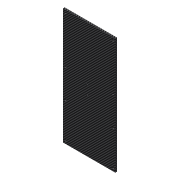
# Autodesk Inventor part: Chassis-2
Saved by Autodesk Inventor 2018 (Build 220112000, 112)
## iProperties
Created: 2018-01-20
Part Number: Chassis-2
Material: CFK
Document SubType Name: Modeling
Designer: fhinstall
Density: 1.43 g/cm^3
Appearance: Kohlenstofffaser
Mass: 68.419 g
Surface Area: 337.638 cm^2
Volume: 47.8454 cm^3
Author: fhinstall
Autodesk Inventor part; units mm, degrees
ref_plane "YZ Plane" through (0, 0, 0) normal (1, 0, 0) x (0, 1, 0)
ref_plane "XZ Plane" through (0, 0, 0) normal (0, 1, 0) x (-1, 0, 0)
ref_plane "XY Plane" through (0, 0, 0) normal (0, 0, 1) x (1, 0, 0)
sketch "Skizze1" plane through (0, 0, 0) normal (0, 1, 0) x (-1, 0, 0)
  line L0 (45, 100) -> (45, -100)
  line L1 (45, -100) -> (-45, -100)
  line L2 (-45, -100) -> (-45, 100)
  line L3 (-45, 100) -> (45, 100)
  line L4 (0, 61.8387) -> (0, -129.7607) construction
  line L5 (83.0665, 0) -> (-88.5254, 0) construction
  circle A0 centre (41, 95) radius 1.7
  circle A1 centre (-41, 95) radius 1.7
  circle A2 centre (-41, -95) radius 1.7
  circle A3 centre (41, -95) radius 1.7
  circle A4 centre (3.1127, 7.2251) radius 1.5558
  circle A5 centre (3.1127, -8.3324) radius 1.5558
  circle A6 centre (-41, 15) radius 1.7
  circle A7 centre (41, 15) radius 1.7
  circle A8 centre (-41, -65) radius 1.7
  circle A9 centre (41, -65) radius 1.7
  circle A10 centre (-41, -145) radius 1.7
  circle A11 centre (41, -145) radius 1.7
  circle A12 centre (-41, -225) radius 1.7
  circle A13 centre (41, -225) radius 1.7
  circle A14 centre (-41, -305) radius 1.7
  circle A15 centre (41, -305) radius 1.7
  circle A16 centre (-41, -385) radius 1.7
  circle A17 centre (41, -385) radius 1.7
  circle A18 centre (-41, -465) radius 1.7
  circle A19 centre (41, -465) radius 1.7
  circle A20 centre (-41, -545) radius 1.7
  circle A21 centre (41, -545) radius 1.7
  circle A22 centre (-41, -625) radius 1.7
  circle A23 centre (41, -625) radius 1.7
  circle A24 centre (-41, -705) radius 1.7
  circle A25 centre (41, -705) radius 1.7
  circle A26 centre (-41, -785) radius 1.7
  circle A27 centre (41, -785) radius 1.7
  circle A28 centre (-41, -865) radius 1.7
  circle A29 centre (41, -865) radius 1.7
  circle A30 centre (-41, -945) radius 1.7
  circle A31 centre (41, -945) radius 1.7
  circle A32 centre (-41, -1025) radius 1.7
  circle A33 centre (41, -1025) radius 1.7
  circle A34 centre (-41, -1105) radius 1.7
  circle A35 centre (41, -1105) radius 1.7
  circle A36 centre (-41, -1185) radius 1.7
  circle A37 centre (41, -1185) radius 1.7
  circle A38 centre (-41, -1265) radius 1.7
  circle A39 centre (41, -1265) radius 1.7
  circle A40 centre (-41, -1345) radius 1.7
  circle A41 centre (41, -1345) radius 1.7
  circle A42 centre (-41, -1425) radius 1.7
  circle A43 centre (41, -1425) radius 1.7
  circle A44 centre (-41, -1505) radius 1.7
  circle A45 centre (41, -1505) radius 1.7
  circle A46 centre (-41, -1585) radius 1.7
  circle A47 centre (41, -1585) radius 1.7
  circle A48 centre (-41, -1665) radius 1.7
  circle A49 centre (41, -1665) radius 1.7
  circle A50 centre (-41, -1745) radius 1.7
  circle A51 centre (41, -1745) radius 1.7
  circle A52 centre (-41, -1825) radius 1.7
  circle A53 centre (41, -1825) radius 1.7
  circle A54 centre (-41, -1905) radius 1.7
  circle A55 centre (41, -1905) radius 1.7
  circle A56 centre (-41, -1985) radius 1.7
  circle A57 centre (41, -1985) radius 1.7
  circle A58 centre (-41, -2065) radius 1.7
  circle A59 centre (41, -2065) radius 1.7
  circle A60 centre (-41, -2145) radius 1.7
  circle A61 centre (41, -2145) radius 1.7
  circle A62 centre (-41, -2225) radius 1.7
  circle A63 centre (41, -2225) radius 1.7
  circle A64 centre (-41, -2305) radius 1.7
  circle A65 centre (41, -2305) radius 1.7
  circle A66 centre (-41, -2385) radius 1.7
  circle A67 centre (41, -2385) radius 1.7
  circle A68 centre (-41, -2465) radius 1.7
  circle A69 centre (41, -2465) radius 1.7
  circle A70 centre (-41, -2545) radius 1.7
  circle A71 centre (41, -2545) radius 1.7
  circle A72 centre (-41, -2625) radius 1.7
  circle A73 centre (41, -2625) radius 1.7
  circle A74 centre (-41, -2705) radius 1.7
  circle A75 centre (41, -2705) radius 1.7
  circle A76 centre (-41, -2785) radius 1.7
  circle A77 centre (41, -2785) radius 1.7
  circle A78 centre (-41, -2865) radius 1.7
  circle A79 centre (41, -2865) radius 1.7
  circle A80 centre (-41, -2945) radius 1.7
  circle A81 centre (41, -2945) radius 1.7
  circle A82 centre (-41, -3025) radius 1.7
  circle A83 centre (41, -3025) radius 1.7
  circle A84 centre (-41, -3105) radius 1.7
  circle A85 centre (41, -3105) radius 1.7
  circle A86 centre (-41, -3185) radius 1.7
  circle A87 centre (41, -3185) radius 1.7
  circle A88 centre (-41, -3265) radius 1.7
  circle A89 centre (41, -3265) radius 1.7
  circle A90 centre (-41, -3345) radius 1.7
  circle A91 centre (41, -3345) radius 1.7
  circle A92 centre (-41, -3425) radius 1.7
  circle A93 centre (41, -3425) radius 1.7
  circle A94 centre (-41, -3505) radius 1.7
  circle A95 centre (41, -3505) radius 1.7
  circle A96 centre (-41, -3585) radius 1.7
  circle A97 centre (41, -3585) radius 1.7
  circle A98 centre (-41, -3665) radius 1.7
  circle A99 centre (41, -3665) radius 1.7
  circle A100 centre (-41, -3745) radius 1.7
  circle A101 centre (41, -3745) radius 1.7
  circle A102 centre (-41, -3825) radius 1.7
  circle A103 centre (41, -3825) radius 1.7
  circle A104 centre (-41, -3905) radius 1.7
  circle A105 centre (41, -3905) radius 1.7
  circle A106 centre (-41, -3985) radius 1.7
  circle A107 centre (41, -3985) radius 1.7
  circle A108 centre (-41, -4065) radius 1.7
  circle A109 centre (41, -4065) radius 1.7
  circle A110 centre (-41, -4145) radius 1.7
  circle A111 centre (41, -4145) radius 1.7
  circle A112 centre (-41, -4225) radius 1.7
  circle A113 centre (41, -4225) radius 1.7
  circle A114 centre (-41, -4305) radius 1.7
  circle A115 centre (41, -4305) radius 1.7
  circle A116 centre (-41, -4385) radius 1.7
  circle A117 centre (41, -4385) radius 1.7
  circle A118 centre (-41, -4465) radius 1.7
  circle A119 centre (41, -4465) radius 1.7
  circle A120 centre (-41, -4545) radius 1.7
  circle A121 centre (41, -4545) radius 1.7
  circle A122 centre (-41, -4625) radius 1.7
  circle A123 centre (41, -4625) radius 1.7
  circle A124 centre (-41, -4705) radius 1.7
  circle A125 centre (41, -4705) radius 1.7
  circle A126 centre (-41, -4785) radius 1.7
  circle A127 centre (41, -4785) radius 1.7
  circle A128 centre (-41, -4865) radius 1.7
  circle A129 centre (41, -4865) radius 1.7
  circle A130 centre (-41, -4945) radius 1.7
  circle A131 centre (41, -4945) radius 1.7
  circle A132 centre (-41, -5025) radius 1.7
  circle A133 centre (41, -5025) radius 1.7
  circle A134 centre (-41, -5105) radius 1.7
  circle A135 centre (41, -5105) radius 1.7
  circle A136 centre (-41, -5185) radius 1.7
  circle A137 centre (41, -5185) radius 1.7
  circle A138 centre (-41, -5265) radius 1.7
  circle A139 centre (41, -5265) radius 1.7
  circle A140 centre (-41, -5345) radius 1.7
  circle A141 centre (41, -5345) radius 1.7
  circle A142 centre (-41, -5425) radius 1.7
  circle A143 centre (41, -5425) radius 1.7
  circle A144 centre (-41, -5505) radius 1.7
  circle A145 centre (41, -5505) radius 1.7
  circle A146 centre (-41, -5585) radius 1.7
  circle A147 centre (41, -5585) radius 1.7
  circle A148 centre (-41, -5665) radius 1.7
  circle A149 centre (41, -5665) radius 1.7
  circle A150 centre (-41, -5745) radius 1.7
  circle A151 centre (41, -5745) radius 1.7
  circle A152 centre (-41, -5825) radius 1.7
  circle A153 centre (41, -5825) radius 1.7
  circle A154 centre (-41, -5905) radius 1.7
  circle A155 centre (41, -5905) radius 1.7
  circle A156 centre (-41, -5985) radius 1.7
  circle A157 centre (41, -5985) radius 1.7
  circle A158 centre (-41, -6065) radius 1.7
  circle A159 centre (41, -6065) radius 1.7
  circle A160 centre (-41, -6145) radius 1.7
  circle A161 centre (41, -6145) radius 1.7
  circle A162 centre (-41, -6225) radius 1.7
  circle A163 centre (41, -6225) radius 1.7
  circle A164 centre (-41, -35) radius 1.7
  circle A165 centre (41, -35) radius 1.7
  point P0 (0, 0)
  dimension "d1" = 45
  dimension "d2" = 45
  dimension "d3" = 100
  dimension "d4" = 100
  dimension "d7" = 3.4
  dimension "d8" = 4
  dimension "d9" = 5
  dimension "d10" = 3.4
  dimension "d11" = 4
  dimension "d12" = 5
  dimension "d13" = 3.4
  dimension "d14" = 4
  dimension "d15" = 5
  dimension "d16" = 3.4
  dimension "d17" = 5
  dimension "d18" = 4
  dimension "d25" = 80
  dimension "d32" = 50
  constraints: 166 centre point, 12 end point, 4 vertical, 2 perpendicular, 2 point on line, 1 horizontal, 324 other
  measures "d1" distance between parallel lines of L0 L4
  measures "d2" distance between parallel lines of L2 L4
  measures "d3" distance between parallel lines of L5 L3
  measures "d4" distance between parallel lines of L5 L1
  measures "d7" diameter of A0
  measures "d8" distance from line of L0 A0.centre
  measures "d9" distance from line of L3 A0.centre
  measures "d10" diameter of A1
  measures "d11" distance from line of L2 A1.centre
  measures "d12" distance from line of L3 A1.centre
  measures "d13" diameter of A2
  measures "d14" distance from line of L2 A2.centre
  measures "d15" distance from line of L1 A2.centre
  measures "d16" diameter of A3
  measures "d17" distance from line of L1 A3.centre
  measures "d18" distance from line of L0 A3.centre
  measures "d25" distance of A1.centre A6.centre
  measures "d32" distance of A6.centre A164.centre
extrude "Extrusion1" add sketch "Skizze1" along normal blind 3 contours L0 L1 L2 L3 | A0 | A1 | A2 | A3 | A4 | A5 | A6 | A7 | A8 | A9 | A164 | A165
extrude "Extrusion2" cut sketch "Skizze1" along normal blind 10 contours A0 | A1 | A2 | A3 | A6 | A7 | A164 | A165
sketch "Skizze2" plane through (0, 0, 0) normal (0, -1, 0) x (1, 0, 0)
  circle A0 centre (1.8873, 7.2251) radius 1.5557 projected
  circle A1 centre (1.8873, -8.3324) radius 1.5557 projected
  point P0 (0, 0)
extrude "Extrusion3" cut sketch "Skizze2" against normal blind 10
